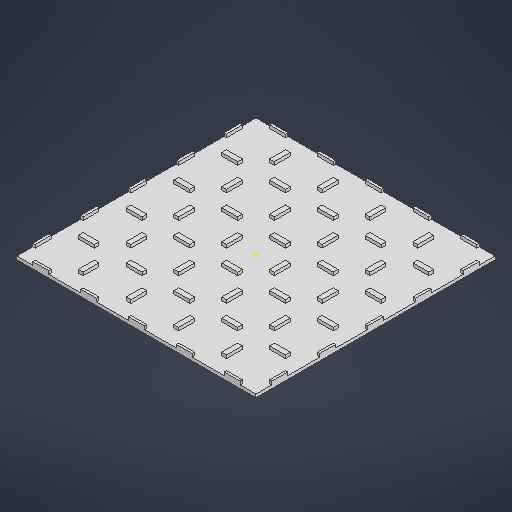
# Autodesk Inventor part: Part3
Saved by Autodesk Inventor 2025.1 (Build 291241000, 241)
## iProperties
Created: 2025-02-19
Part Number: Part3
Material: Generic
Document SubType Name: Modeling
Designer: jerem
Density: 1 g/cm^3
Appearance: Default
Author: jerem
Autodesk Inventor part; units mm, degrees
ref_plane "YZ Plane" through (0, 0, 0) normal (1, 0, 0) x (0, 1, 0)
ref_plane "XZ Plane" through (0, 0, 0) normal (0, 1, 0) x (-1, 0, 0)
ref_plane "XY Plane" through (0, 0, 0) normal (0, 0, 1) x (1, 0, 0)
sketch "Sketch1" plane through (0, 0, 0) normal (0, 1, 0) x (-1, 0, 0)
  line L0 (-15, -15) -> (15, -15)
  line L1 (15, -15) -> (15, 15)
  line L2 (15, 15) -> (-15, 15)
  line L3 (-15, 15) -> (-15, -15)
  line L4 (-15, -15) -> (15, 15) construction
  line L5 (15, -15) -> (-15, 15) construction
  line L6 (15, 5) -> (13.5, 5)
  line L7 (13.5, 5) -> (13.5, -5)
  line L8 (13.5, -5) -> (15, -5)
  line L9 (13.5, 0) -> (15, 0) construction
  line L10 (5, 15) -> (5, 13.5)
  line L11 (5, 13.5) -> (-5, 13.5)
  line L12 (-5, 13.5) -> (-5, 15)
  line L13 (-5, -15) -> (-5, -13.5)
  line L14 (-5, -13.5) -> (5, -13.5)
  line L15 (5, -13.5) -> (5, -15)
  line L16 (-15, -5) -> (-13.5, -5)
  line L17 (-13.5, -5) -> (-13.5, 5)
  line L18 (-13.5, 5) -> (-15, 5)
  line L19 (-12.7, -12.7) -> (12.7, -12.7) construction
  line L20 (12.7, -12.7) -> (12.7, 12.7) construction
  line L21 (12.7, 12.7) -> (-12.7, 12.7) construction
  line L22 (-12.7, 12.7) -> (-12.7, -12.7) construction
  line L23 (-12.7, -12.7) -> (12.7, 12.7) construction
  line L24 (12.7, -12.7) -> (-12.7, 12.7) construction
  point P0 (0, 0)
  point P1 (12.7, 0)
  dimension "d0" = 30
  dimension "d3" = 10
  dimension "d8" = 25.4
  dimension "d10" = 27
  constraints: 50 end point, 12 symmetric about line, 7 midpoint, 4 equal length, 4 parallel, 4 perpendicular, 3 horizontal, 2 point on line, 1 vertical
  measures "d0" distance of L2.end L1.end
  measures "d3" distance of L6.end L7.end
  measures "d8" distance of L21.end L20.end
  measures "d10" distance between parallel lines of L17 L7
extrude "Extrusion1" add sketch "Sketch1" against normal blind 2
extrude "Extrusion2" add sketch "Sketch1" along normal blind 2 contours L13 L14 L15 L0 | L3 L18 L17 L16 | L8 L7 L6 L1 | L2 L10 L11 L12
pattern_linear "Rectangular Pattern1" count 5 spacing 30 along (0, 0, 1) count 5 spacing 30 along (1, 0, 0) of "Extrusion1", "Extrusion2" first direction both ways yes second direction both ways yes
sketch "Sketch2" plane through (0, 0, 0) normal (0, 1, 0) x (1, 0, 0)
  point P0 (0, 0)
body "Solid1"
